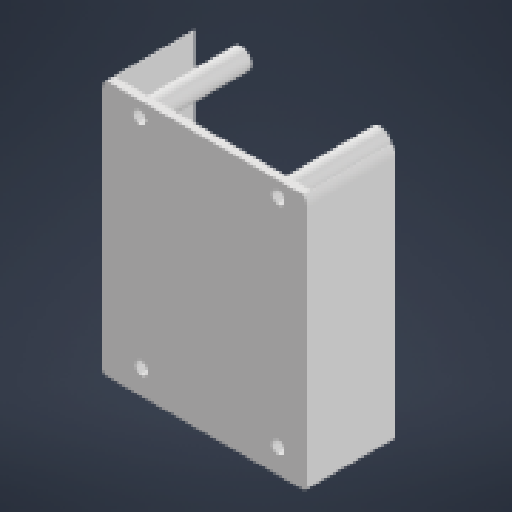
# Autodesk Inventor part: case-top
Saved by Autodesk Inventor 2026.2 (Build 302298000, 298)
## iProperties
Created: 2026-05-31
Part Number: case-top
Material: Generic
Document SubType Name: Modeling
Designer: FromDarkHell
Density: 1 g/cm^3
Appearance: Default
Author: FromDarkHell
Autodesk Inventor part; units mm, degrees
ref_plane "YZ Plane" through (0, 0, 0) normal (1, 0, 0) x (0, 1, 0)
ref_plane "XZ Plane" through (0, 0, 0) normal (0, 1, 0) x (-1, 0, 0)
sketch "Sketch1" plane through (0, 0, 0) normal (0, 0, 1) x (1, 0, 0)
  circle A0 centre (-41.65, 59.825) radius 1.6 projected
  circle A1 centre (-41.15, 6.075) radius 1.6 projected
  circle A2 centre (-7.15, 59.825) radius 1.6 projected
  circle A3 centre (-7.15, 6.075) radius 1.6 projected
  line L0 (-1, 63.5) -> (-1, 0) projected
  line L1 (-1, 63.5) -> (-49.8, 63.5) projected
  line L2 (-49.8, 0) -> (-49.8, 63.5) projected
  line L3 (-1, 0) -> (-49.8, 0) projected
  ellipse E0 centre (-49.8, 61.0858) end of major axis (-49.8, 63.5) minor radius 1 (-49.8, 63.5) -> (-50.8, 61.0858) ccw projected
  line L4 (-50.8, 61.0858) -> (-50.8, 1) projected
  arc A4 (-50.8, 1) -> (-49.8, 0) centre (-49.8, 1) ccw projected
  arc A5 (-1, 0) -> (0, 1) centre (-1, 1) ccw projected
  line L5 (0, 1) -> (0, 61.0858) projected
  ellipse E1 centre (-1, 61.0858) end of major axis (-1, 58.6716) minor radius 1 (0, 61.0858) -> (-1, 63.5) ccw projected
  line L6 (-48.9, 5.825) -> (-48.9, 59.5) projected
  arc A6 (-44.9, 63.5) -> (-48.9, 59.5) centre (-44.9, 59.5) ccw projected
  arc A7 (-1.9, 59.5) -> (-5.9, 63.5) centre (-5.9, 59.5) ccw projected
  line L7 (-1.9, 59.5) -> (-1.9, 5.825) projected
  arc A8 (-48.9, 5.825) -> (-44.9, 1.825) centre (-44.9, 5.825) ccw projected
  line L8 (-5.9, 1.825) -> (-44.9, 1.825) projected
  arc A9 (-5.9, 1.825) -> (-1.9, 5.825) centre (-5.9, 5.825) ccw projected
  line L9 (-49.8, 1) -> (-1, 1)
  point P0 (0, 0)
  constraints: 2 end point, 1 parallel, 2 other
extrude "Extrusion1" add sketch "Sketch1" along normal blind 20 contours E1 L5 A5 L0 | L0 L3 L2 L9 | L2 A4 L4 E0
sketch "Sketch2" plane through (0, 0, 20) normal (0, 0, 1) x (1, 0, 0)
  line L0 (-1, 63.5) -> (-49.8, 63.5) projected
  ellipse E0 centre (-49.8, 61.0858) end of major axis (-49.8, 63.5) minor radius 1 (-49.8, 63.5) -> (-50.8, 61.0858) ccw projected
  line L1 (-49.8, 0) -> (-1, 0) projected
  arc A0 (-1, 0) -> (0, 1) centre (-1, 1) ccw projected
  line L2 (0, 1) -> (0, 61.0858) projected
  ellipse E1 centre (-1, 61.0858) end of major axis (-1, 58.6716) minor radius 1 (0, 61.0858) -> (-1, 63.5) ccw projected
  line L3 (-1, 63.5) -> (-1, 1) projected
  line L4 (-1, 1) -> (-49.8, 1) projected
  line L5 (-49.8, 1) -> (-49.8, 63.5) projected
  ellipse E2 centre (-49.8, 61.0858) end of major axis (-49.8, 63.5) minor radius 1 (-49.8, 63.5) -> (-50.8, 61.0858) ccw projected
  line L6 (-50.8, 61.0858) -> (-50.8, 1) projected
  arc A1 (-50.8, 1) -> (-49.8, 0) centre (-49.8, 1) ccw projected
  arc A2 (-44.9, 63.5) -> (-48.9, 59.5) centre (-44.9, 59.5) ccw projected
  arc A3 (-1.9, 59.5) -> (-5.9, 63.5) centre (-5.9, 59.5) ccw projected
  line L7 (-48.9, 59.5) -> (-49.8, 59.5)
  line L8 (-1.9, 59.5) -> (-1, 59.5)
  line L9 (-1.9, 59.5) -> (-48.9, 59.5)
  line L10 (-5.9, 1.825) -> (-44.9, 1.825) projected
  line L11 (-44.9, 1.825) -> (-49.8, 1.825)
  line L12 (-5.9, 1.825) -> (-1, 1.825)
  point P0 (0, 0)
  constraints: 10 end point, 6 point on line, 2 perpendicular, 1 collinear, 3 other
extrude "Extrusion2" add sketch "Sketch2" along normal blind 2
sketch "Sketch3" plane through (0, 0, 22) normal (0, 0, 1) x (1, 0, 0)
  circle A0 centre (-41.65, 59.825) radius 1.6 projected
  circle A1 centre (-7.15, 59.825) radius 1.6 projected
  circle A2 centre (-7.15, 6.075) radius 1.6 projected
  circle A3 centre (-41.15, 6.075) radius 1.6 projected
  point P0 (0, 0)
extrude "Extrusion3" cut sketch "Sketch3" against normal through all
ref_plane "Work Plane1" through (-49.495, 1.3716, 1.51) normal (0, 0, 1) x (1, 0, 0)
sketch "Sketch4" plane through (0, 0, 22) normal (0, 0, 1) x (1, 0, 0)
  circle A0 centre (-41.65, 59.825) radius 1.6 projected
  circle A1 centre (-41.15, 6.075) radius 1.6 projected
  circle A2 centre (-7.15, 6.075) radius 1.6 projected
  circle A3 centre (-7.15, 59.825) radius 1.6 projected
  circle A4 centre (-41.65, 59.825) radius 2.6
  circle A5 centre (-7.15, 59.825) radius 2.6
  circle A6 centre (-7.15, 6.075) radius 2.6
  circle A7 centre (-41.15, 6.075) radius 2.6
  point P0 (0, 0)
  dimension "d10" = 1
  dimension "d11" = 1
  dimension "d12" = 1
  dimension "d13" = 1
  constraints: 4 centre point
  measures "d10" radial gap between concentric circles of A0 A4
  measures "d11" radial gap between concentric circles of A3 A5
  measures "d12" radial gap between concentric circles of A2 A6
  measures "d13" radial gap between concentric circles of A1 A7
extrude "Extrusion4" add sketch "Sketch4" against normal up to surface (20.49 mm away)
body "Solid1"
